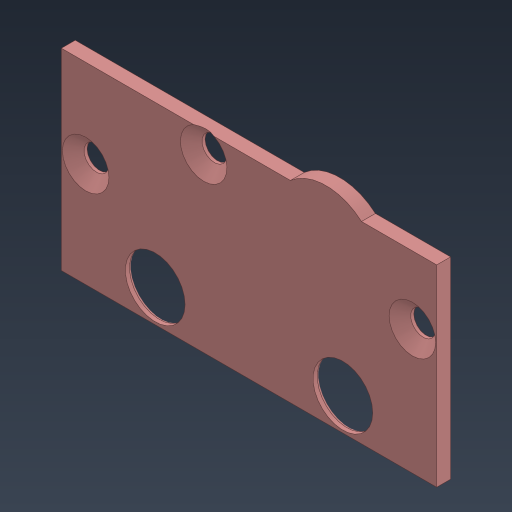
# Autodesk Inventor part: gearbox-wall-right
Saved by Autodesk Inventor 2023 (Build 270158000, 158)
## iProperties
Created: 2025-04-19
Part Number: gearbox-wall-right
Material: Generic
Document SubType Name: Modeling
Designer: szymo
Density: 1 g/cm^3
Appearance: Default(1)
Mass: 2.54755 g
Surface Area: 31.7059 cm^2
Volume: 2.54755 cm^3
Author: szymo
Autodesk Inventor part; units mm, degrees
ref_plane "YZ Plane" through (0, 0, 0) normal (1, 0, 0) x (0, 1, 0)
ref_plane "XZ Plane" through (0, 0, 0) normal (0, 1, 0) x (-1, 0, 0)
ref_plane "XY Plane" through (0, 0, 0) normal (0, 0, 1) x (1, 0, 0)
sketch "Sketch1" plane through (0, 0, 0) normal (0, 0, 1) x (1, 0, 0)
  arc A0 (-6.2914, -1.7988) -> (-23.3552, -14.6314) centre (-13.5, -9.9747) ccw projected
  arc A1 (23.3552, -14.6314) -> (19.9355, -1.1773) centre (13.5, -9.9747) ccw projected
  line L0 (-27, -14.6314) -> (-23.3552, -14.6314) projected
  line L1 (-27, 13.0686) -> (27, 13.0686)
  line L2 (27, 13.0686) -> (27, -14.6314)
  line L3 (27, -14.6314) -> (-27, -14.6314)
  line L4 (-27, -14.6314) -> (-27, 13.0686)
  circle A2 centre (-13.5, -9.9747) radius 6 projected
  circle A3 centre (13.5, -9.9747) radius 6 projected
  circle A4 centre (-13.5, -9.9747) radius 6.3
  circle A5 centre (13.5, -9.9747) radius 6.3
  circle A6 centre (-23.5, 0.3867) radius 2.5 projected
  circle A7 centre (23.5, 3.3227) radius 2.5 projected
  circle A8 centre (-6.5264, 10.0686) radius 2.5 projected
  arc A9 (-2.7267, 0.5805) -> (-6.2914, -1.7988) centre (0, -7.3647) ccw projected
  arc A10 (4.0839, 8.7878) -> (-2.7267, 0.5805) centre (4.344, 1.6425) ccw projected
  arc A11 (17.3504, 3.8358) -> (4.0839, 8.7878) centre (11.0654, 7.2448) ccw projected
  arc A12 (19.9355, -1.1773) -> (17.3504, 3.8358) centre (14.55, -0.7814) ccw projected
  line L5 (23.3552, -14.6314) -> (27, -14.6314) projected
  line L6 (27, -14.6314) -> (27, 13.0686) projected
  line L7 (27, 13.0686) -> (16.1787, 13.0686) projected
  arc A13 (16.1787, 13.0686) -> (5.9521, 13.0686) centre (11.0654, 7.2448) ccw projected
  line L8 (5.9521, 13.0686) -> (-27, 13.0686) projected
  line L9 (-27, 13.0686) -> (-27, -14.6314) projected
  point P0 (0, 0)
  point P1 (-17.7433, -14.6314)
  point P2 (-9.2567, -14.6314)
  point P3 (9.2567, -14.6314)
  point P4 (17.7433, -14.6314)
  point P5 (23.3552, -14.6314)
  point P6 (15.2134, 13.0686)
  point P7 (6.9174, 13.0686)
  point P8 (-23.3552, -14.6314)
  point P9 (5.9521, 13.0686)
  point P10 (-23.3552, -14.6314)
  point P11 (9.7164, -14.6314)
  point P12 (17.2836, -14.6314)
  dimension "d0" = 0.3
  dimension "d1" = 0.3
  constraints: 8 end point, 2 centre point, 2 parallel, 1 horizontal, 1 perpendicular
  measures "d0" radial gap between concentric circles of A2 A4
  measures "d1" radial gap between concentric circles of A3 A5
ref_plane "Work Plane1" through (-19.5, -15.9747, 1) normal (0, 0, 1) x (1, 0, 0)
extrude "Extrusion1" add sketch "Sketch1" along normal up to surface (1 mm away) contours A9 A10 A11 L1 A12 A1 L3 A5 A4 A0 | A0 L0 L4 L1 A11 A10 A9 | A11 L1 | L1 A13 A11 | A5 L3 A3 | L1 L2 L3 A1 A12 A11 | A6 | A7 | A8 picked at (7.9397, -7.5351)
sketch "Sketch2" plane through (-27, 13.0686, 1) normal (0, 0, 1) x (1, 0, 0)
  line L0 (54, 0) -> (54, -27.7) projected
  line L1 (43.1787, 0) -> (54, 0) projected
  line L2 (0, -27.7) -> (0, 0) projected
  line L3 (9.2567, -27.7) -> (0, -27.7) projected
  circle A0 centre (13.5, -23.0433) radius 4 projected
  circle A1 centre (40.5, -23.0433) radius 4 projected
  circle A2 centre (13.5, -23.0433) radius 4.3
  circle A3 centre (40.5, -23.0433) radius 4.3
  line L4 (9.2567, -27.7) -> (17.7433, -27.7)
  line L5 (0, -27.7) -> (54, -27.7) projected
  line L6 (36.2567, -27.7) -> (44.7433, -27.7)
  line L7 (0, 0) -> (32.9521, 0) projected
  arc A4 (43.1787, 0) -> (32.9521, 0) centre (38.0654, -5.8238) ccw projected
  arc A5 (17.7433, -27.7) -> (9.2567, -27.7) centre (13.5, -23.0433) ccw projected
  line L8 (36.7164, -27.7) -> (17.7433, -27.7) projected
  arc A6 (44.2836, -27.7) -> (36.7164, -27.7) centre (40.5, -23.0433) ccw projected
  line L9 (54, -27.7) -> (44.2836, -27.7) projected
  point P0 (27, -13.0686)
  point P1 (36.7164, -27.7)
  point P2 (44.2836, -27.7)
  point P3 (17.7433, -27.7)
  dimension "d4" = 0.3
  dimension "d5" = 0.3
  constraints: 4 end point, 2 centre point, 1 collinear
  measures "d4" radial gap between concentric circles of A0 A2
  measures "d5" radial gap between concentric circles of A1 A3
ref_plane "Work Plane2" through (-17.5, -13.9747, 2) normal (0, 0, 1) x (1, 0, 0)
extrude "Extrusion2" add sketch "Sketch2" along normal up to surface (1 mm away) contours L0 L5 A6 A5 L3 L2 L7 A4 L1 | L5 A6 | A5 L4
sketch "Sketch3" plane through (-27, -14.6314, 2) normal (0, 0, 1) x (1, 0, 0)
  circle A0 centre (3.5, 15.0181) radius 2.5 projected
  circle A1 centre (50.5, 17.9541) radius 2.5 projected
  circle A2 centre (20.4736, 24.7) radius 2.5 projected
  arc A3 (20.7086, 12.8326) -> (3.6448, 0) centre (13.5, 4.6567) ccw projected
  arc A4 (50.3552, 0) -> (46.9355, 13.4541) centre (40.5, 4.6567) ccw projected
  line L0 (0, 0) -> (3.6448, 0) projected
  arc A5 (24.2733, 15.2119) -> (20.7086, 12.8326) centre (27, 7.2667) ccw projected
  arc A6 (31.0839, 23.4192) -> (24.2733, 15.2119) centre (31.344, 16.2739) ccw projected
  arc A7 (44.3504, 18.4671) -> (31.0839, 23.4192) centre (38.0654, 21.8762) ccw projected
  arc A8 (46.9355, 13.4541) -> (44.3504, 18.4671) centre (41.55, 13.85) ccw projected
  line L1 (50.3552, 0) -> (54, 0) projected
  line L2 (54, 0) -> (54, 27.7) projected
  line L3 (54, 27.7) -> (43.1787, 27.7) projected
  arc A9 (43.1787, 27.7) -> (32.9521, 27.7) centre (38.0654, 21.8762) ccw projected
  line L4 (32.9521, 27.7) -> (0, 27.7) projected
  line L5 (0, 27.7) -> (0, 0) projected
  point P0 (27, 14.6314)
  point P1 (3.5, 15.0181)
  point P2 (50.5, 17.9541)
  constraints: 3 coincident
hole "Hole1" at (-23.5, 0.3867, 2) at (-6.5264, 10.0686, 2) at (23.5, 3.3227, 2) direction (0, 0, -1) diameter 3.6 depth 5 countersink diameter 6.7 countersink angle 90 clearance for "Countersunk Flat Head Screw ISO 2009/7046" size "M3" standard "ISO"
fillet "Fillet1" radius 0.4 3 edges at (9.2, -9.9747, 1) (-13.5, -3.6747, 0) (-17.8, -9.9747, 1)
sketch "Sketch4" plane through (0, 0, 0) normal (0, 0, -1) x (-1, 0, 0)
  circle A0 centre (0, -7.3647) radius 1.25 projected
  circle A1 centre (-4.344, 1.6425) radius 1.25 projected
  circle A2 centre (-11.0654, 7.2448) radius 1.25 projected
  circle A3 centre (-11.0654, 7.2448) radius 1.45
  circle A4 centre (-4.344, 1.6425) radius 1.45
  circle A5 centre (0, -7.3647) radius 1.45
  point P0 (0, 0)
  dimension "d16" = 0.2
  dimension "d17" = 0.2
  dimension "d18" = 0.2
  constraints: 3 centre point
  measures "d16" radial gap between concentric circles of A2 A3
  measures "d17" radial gap between concentric circles of A1 A4
  measures "d18" radial gap between concentric circles of A0 A5
extrude "Extrusion3" cut sketch "Sketch4" against normal blind 1.4 contours A0 | A1 | A2 | A3 | A4 | A5
fillet "Fillet2" radius 0.4 4 edges at (12.5154, 7.2448, 0) (5.794, 1.6425, 0) (1.45, -7.3647, 0) (13.5, -3.9747, 0)
body "Solid1"
